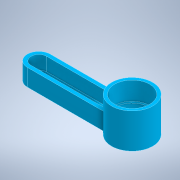
# Autodesk Inventor part: birdWaterForCageAttachement
Saved by Autodesk Inventor 2022.1 (Build 261234020, 234B)
## iProperties
Created: 2021-10-28
Part Number: birdWaterForCageAttachement
Material: ABS Plastic
Document SubType Name: Modeling
Designer: robst
Density: 1.06 g/cm^3
Appearance: Sky Blue Medium
Author: robst
Autodesk Inventor part; units mm, degrees
ref_plane "YZ Plane" through (0, 0, 0) normal (1, 0, 0) x (0, 1, 0)
ref_plane "XZ Plane" through (0, 0, 0) normal (0, 1, 0) x (-1, 0, 0)
ref_plane "XY Plane" through (0, 0, 0) normal (0, 0, 1) x (1, 0, 0)
sketch "Sketch2" plane through (0, 0, 0) normal (0, 1, 0) x (-1, 0, 0)
  line L0 (38.1, 0) -> (-38.1, 0) construction
  line L1 (38.1, 9.35) -> (-24.2025, 9.35)
  line L2 (-24.2025, -9.35) -> (38.1, -9.35)
  arc A0 (38.1, -9.35) -> (38.1, 9.35) centre (38.1, 0) ccw
  line L3 (38.1, 0) -> (-38.1, 0) construction
  line L4 (38.1, 6.35) -> (-22.6003, 6.35)
  line L5 (-22.6003, -6.35) -> (38.1, -6.35)
  arc A1 (38.1, -6.35) -> (38.1, 6.35) centre (38.1, 0) ccw
  circle A2 centre (-38.1, 0) radius 14.25
  circle A3 centre (-38.1, 0) radius 16.75
  point P0 (0, 0)
  point P1 (-32.1033, 12.9268)
  point P2 (-27.8247, 9.8732)
  point P3 (-27.8247, -9.8732)
  point P4 (47.45, 0)
  point P5 (44.45, 0)
  dimension "d20" = 18.7
  dimension "d21" = 76.2
  dimension "d22" = 3
  dimension "d23" = 3
  dimension "d67" = 28.5
  dimension "d68" = 33.5
  constraints: 16 end point, 13 point on circle, 4 centre point, 4 tangent, 2 coincident, 2 midpoint, 2 parallel, 1 horizontal, 1 point on line
  measures "d20" distance between parallel lines of L1 L2
  measures "d21" distance of L0.end L0.start
  measures "d22" distance between parallel lines of L5 L2
  measures "d23" distance of point (47.45, 0) point (44.45, 0)
  measures "d67" diameter of A2
  measures "d68" diameter of A3
extrude "baseExtrsion" add sketch "Sketch2" against normal blind 3 contours A0 L2 A3 L5 A1 L4 L1 | A3 | L4 A1 L5 A3 | A2
extrude "drinkingPortionExtrusion" add sketch "Sketch2" along normal blind 10.97 contours A0 L2 A3 L5 A1 L4 L1
extrude "capExtrusion" add sketch "Sketch2" along normal blind 25.4 contours A3
sketch "Sketch4" plane through (0, 0, 0) normal (0, 1, 0) x (1, 0, 0)
  circle A0 centre (38.1, 0) radius 16.75 projected
  circle A1 centre (38.1, 0) radius 14.25 projected
  line L0 (22.6003, 6.35) -> (-38.1, 6.35) projected
  line L1 (-38.1, -6.35) -> (22.6003, -6.35) projected
  arc A2 (25.343, 6.35) -> (25.343, -6.35) centre (38.1, 0) ccw
  arc A3 (22.6003, 6.35) -> (22.6003, -6.35) centre (38.1, 0) ccw
  line L2 (22.6003, 6.35) -> (-38.1, 6.35) projected
  line L3 (22.6003, 6.35) -> (25.343, 6.35)
  line L4 (-38.1, -6.35) -> (22.6003, -6.35) projected
  line L5 (22.6003, -6.35) -> (25.343, -6.35)
  point P0 (0, 0)
  point P1 (25.343, -6.35)
  point P2 (25.343, 6.35)
  point P3 (-323.7292, -9.35)
  point P4 (-323.7292, 9.35)
  constraints: 4 end point, 4 point on circle, 2 centre point, 2 coincident, 1 concentric, 1 horizontal, 1 parallel, 2 other
extrude "slotForWaterExtrusion" cut sketch "Sketch4" along normal blind 3.175 contours L3 A1 L5 A0 picked at (24.0572, -5.3205)
ref_plane "Work Plane2" through (0, 3.175, 0) normal (0, 1, 0) x (1, 0, 0)
sketch "Sketch6" plane through (0, 3.175, 0) normal (0, 1, 0) x (1, 0, 0)
  arc A0 (25.343, -6.35) -> (25.343, 6.35) centre (38.1, 0) ccw projected
  circle A1 centre (38.1, 0) radius 14.25
  circle A2 centre (38.1, 0) radius 12.5
  point P0 (0, 0)
  point P1 (23.8548, 0.3681)
  point P2 (52.35, 0)
  point P3 (-323.7292, -9.35)
  point P4 (-323.7292, 9.35)
  point P5 (25.343, 6.35)
  point P6 (25.343, -6.35)
  dimension "d72" = 25
  constraints: 2 coincident, 1 centre point, 3 other
  measures "d72" diameter of A2
extrude "Extrusion10" add sketch "Sketch6" along normal blind 7.225
sketch "Sketch7" plane through (0, -3, 0) normal (0, -1, 0) x (1, 0, 0)
  line L0 (-38.1, 0) -> (21.35, 0) construction
  circle A0 centre (38.1, 0) radius 16.75 construction
  point P0 (0, 0)
  constraints: 2 end point, 2 horizontal, 1 horizontal alignment, 1 other
sketch "Sketch5" plane through (0, 0, 0) normal (0, 0, 1) x (1, 0, 0)
  line L0 (52.35, 25.4) -> (52.35, 0) projected
  line L1 (54.85, 25.4) -> (21.35, 25.4) projected
  line L2 (52.35, 25.4) -> (52.35, 31.75) construction
  line L3 (52.35, 0) -> (25.343, 0) construction
  line L4 (52.35, 25.4) -> (52.35, 0) projected
  line L5 (23.85, 25.4) -> (23.85, 3.175) projected
  line L6 (27.333, 0) -> (27.333, 3.175) projected
  line L7 (27.333, 3.175) -> (27.333, 3.175) projected
  line L8 (27.333, 3.175) -> (27.333, 0) projected
  line L9 (27.333, 0) -> (27.333, 0) projected
  line L10 (25.6, 25.4) -> (50.6, 25.4) projected
  line L11 (23.85, 25.4) -> (52.35, 25.4) projected
  line L12 (38.1, 25.4) -> (38.1, 0) construction
  line L13 (52.5078, 30.2794) -> (54.5908, 29.7874)
  line L14 (52.5262, 28.8138) -> (54.6092, 29.3059)
  arc A0 (54.6092, 29.3059) -> (54.5908, 29.7874) centre (54.5333, 29.5441) ccw
  arc A1 (52.35, 30.5118) -> (52.5078, 30.2794) centre (52.6, 30.5118) ccw
  arc A2 (52.5262, 28.8138) -> (52.35, 28.575) centre (52.6, 28.575) ccw
  line L15 (54.5908, 29.7874) -> (52.35, 29.7874) construction
  line L16 (54.6092, 29.3059) -> (52.35, 29.3059) construction
  line L17 (52.35, 30.5118) -> (52.35, 28.575) construction
  line L18 (52.35, 30.5118) -> (52.35, 28.575)
  line L19 (54.85, 25.4) -> (54.85, -3) projected
  point P0 (0, 0)
  point P1 (54.7831, 29.5536)
  dimension "d34" = 6.35
  dimension "d35" = 3.175
  dimension "d56" = 0.25
  dimension "d62" = 26.58
  dimension "d64" = 3.175
  dimension "d66" = 2.4331
  constraints: 16 end point, 7 point on circle, 4 point on line, 4 tangent, 3 centre point, 3 midpoint, 3 perpendicular, 2 collinear, 1 equal length, 1 equal radius, 1 vertical
  measures "d34" distance of L0.start L2.end
  measures "d35" distance of point (52.35, 28.575) L0.start
  measures "d56" radius of A0
  measures "d62" angle of L13 L14
  measures "d64" distance from line of L17.end L1
  measures "d66" horizontal distance of point (54.783, 29.554) L15.end
equation "\"d20\" = baseExteriorWidth"
equation "\"d21\" = baseLength"
equation "\"d22\" = baseWallThickness"
equation "\"d23\" = baseWallThickness"
equation "\"d67\" = capInteriorDiameter"
equation "\"d68\" = capExteriorDiameter"
equation "\"d24\" = baseWallThickness"
equation "\"d26\" = baseHeight - baseWallThickness"
equation "\"d28\" = capHeight"
equation "\"d30\" = heightForWaterSlot"
equation "\"d72\" = diameterOfShelf"
equation "\"d73\" = -heightForWaterSlot + capHeight - heigthForBottleCap"
equation "\"baseLength\" = 76.2"
equation "\"baseExteriorWidth\" = baseInteriorWidth + 2 * baseWallThickness"
equation "\"baseHeight\" = 13.97"
equation "\"capInteriorDiameter\" = 28.5"
equation "\"capWallThickness\" = 2.5"
equation "\"capExteriorDiameter\" = capInteriorDiameter + 2 * capWallThickness"
equation "\"baseWallThickness\" = 3"
equation "\"capHeight\" = 25.4"
equation "\"heightForWaterSlot\" = 3.175"
equation "\"baseInteriorWidth\" = 12.7"
equation "\"d69\" = heightForWaterSlot"
equation "\"diameterOfShelf\" = 25"
equation "\"heigthForBottleCap\" = 15"
body "Solid1"
body "Solid2"
